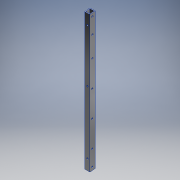
# Autodesk Inventor part: Turret Support Extrusion
Saved by Autodesk Inventor 2019.4 (Build 234330000, 330)
## iProperties
Created: 2020-01-11
Part Number: Turret Support Extrusion
Material: Aluminum 6061
Document SubType Name: Modeling
Designer: admin
Density: 2.7 g/cm^3
Appearance: Aluminum - Flat
Author: admin
Autodesk Inventor part; units mm, degrees
ref_plane "YZ Plane" through (0, 0, 0) normal (1, 0, 0) x (0, 1, 0)
ref_plane "XZ Plane" through (0, 0, 0) normal (0, 1, 0) x (-1, 0, 0)
ref_plane "XY Plane" through (0, 0, 0) normal (0, 0, 1) x (1, 0, 0)
sketch "Sketch1" plane through (0, 0, 0) normal (0, 1, 0) x (-1, 0, 0)
  line L0 (-10, 10) -> (10, 10)
  line L1 (10, 10) -> (10, -10)
  line L2 (10, -10) -> (-10, -10)
  line L3 (-10, -10) -> (-10, 10)
  line L4 (-10, 10) -> (10, -10) construction
  line L5 (10, 10) -> (-10, -10) construction
  line L6 (8, -8) -> (8, 8)
  line L7 (8, 8) -> (-8, 8)
  line L8 (-8, 8) -> (-8, -8)
  line L9 (-8, -8) -> (8, -8)
  point P0 (0, 0)
  dimension "d0" = 20
  dimension "d1" = 20
  dimension "d2" = 2
  constraints: 20 end point, 4 parallel, 2 midpoint, 2 perpendicular, 1 horizontal, 3 other
  measures "d0" distance of L1.end L2.end
  measures "d1" distance of L0.end L1.end
  measures "d2" distance between parallel lines of L1 L6
extrude "Extrusion1" add sketch "Sketch1" along normal blind 550
sketch "Sketch2" plane through (10, 0, 10) normal (1, 0, 0) x (0, 0, -1)
  line L0 (0, 0) -> (0, 550) projected
  line L1 (0, 0) -> (20, 2.261)
  line L2 (20, 0) -> (20, 550) projected
  line L3 (0, 523.3124) -> (20, 525.5735)
  line L4 (20, 525.5735) -> (78.4148, 8.8649) construction
  line L5 (78.4148, 8.8649) -> (20, 2.261) construction
  line L6 (0, 550) -> (20, 550) projected
  line L7 (20, 0) -> (0, 0) projected
  point P0 (10, 0)
  dimension "d5" = 83.55
  dimension "d6" = 83.55
  dimension "d7" = 520
  constraints: 8 end point, 3 point on line, 1 collinear, 1 perpendicular
  measures "d5" angle of L0 L1
  measures "d6" angle of L0 L3
  measures "d7" distance of L3.end L4.end
extrude "Extrusion2" cut sketch "Sketch2" against normal through all contours L1 L2 L7 | L0 L6 L2 L3
sketch "Sketch3" plane through (10, 2.261, -10) normal (1, 0, 0) x (0, 0, -1)
  line L0 (-11.3735, 10.7907) -> (-10.6994, 510.0264) construction
  line L1 (-20, -2.261) -> (-20, 521.0514) projected
  circle A0 centre (-10.6994, 510.0264) radius 2.75
  circle A1 centre (-11.3735, 10.7907) radius 2.75 projected
  circle A2 centre (-10.6994, 510.0264) radius 2.75 projected
  circle A3 centre (-11.2925, 70.7907) radius 2.75
  circle A4 centre (-11.1574, 170.7907) radius 2.75
  circle A5 centre (-11.0224, 270.7907) radius 2.75
  circle A6 centre (-10.8874, 370.7907) radius 2.75
  circle A7 centre (-10.7804, 450.0264) radius 2.75
  point P0 (-10, -2.261)
  dimension "d11" = 5.5
  dimension "d13" = 5.5
  dimension "d14" = 5.5
  dimension "d15" = 5.5
  dimension "d16" = 5.5
  dimension "d17" = 5.5
  dimension "d18" = 60
  dimension "d19" = 60
  dimension "d20" = 100
  dimension "d21" = 100
  dimension "d22" = 100
  constraints: 6 centre point, 5 point on line, 3 coincident, 2 end point
  measures "d11" diameter of A0
  measures "d13" diameter of A3
  measures "d14" diameter of A4
  measures "d15" diameter of A5
  measures "d16" diameter of A6
  measures "d17" diameter of A7
  measures "d18" distance of A7.centre A0.centre
  measures "d19" distance of A3.centre A1.centre
  measures "d20" distance of A4.centre A3.centre
  measures "d21" distance of A5.centre A4.centre
  measures "d22" distance of A5.centre A6.centre
extrude "Extrusion3" cut sketch "Sketch3" against normal through all
sketch "Sketch4" plane through (-10, 523.3124, 10) normal (0, 0, 1) x (1, 0, 0)
  line L0 (10, -523.3124) -> (10, 0) construction
  line L1 (20, 0) -> (0, 0) projected
  circle A0 centre (10, -40) radius 2.75
  circle A1 centre (10, -483.3124) radius 2.75
  circle A2 centre (10, -243.3124) radius 2.75
  line L2 (20, -523.3124) -> (0, -523.3124) projected
  dimension "d25" = 5.5
  dimension "d26" = 5.5
  dimension "d27" = 5.5
  dimension "d28" = 40
  dimension "d29" = 40
  dimension "d30" = 240
  constraints: 3 centre point, 3 point on line, 2 end point, 1 midpoint
  measures "d25" diameter of A0
  measures "d26" diameter of A1
  measures "d27" diameter of A2
  measures "d28" distance from line of L2 A1.centre
  measures "d29" distance from line of L1 A0.centre
  measures "d30" distance of A1.centre A2.centre
extrude "Extrusion4" cut sketch "Sketch4" against normal through all
body "Solid1"
